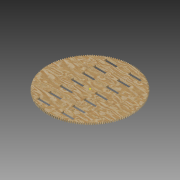
# Autodesk Inventor part: 1228_Major Gear_V1
Saved by Autodesk Inventor 2020 (Build 240168000, 168)
## iProperties
Created: 2019-09-12
Part Number: 1228_Major Gear_V1
Material: Generic
Document SubType Name: Modeling
Designer: MPI
Density: 1 g/cm^3
Appearance: Plywood - Weathered
Mass: 13454.9 g
Surface Area: 16406.6 cm^2
Volume: 13454.9 cm^3
Author: MPI
Autodesk Inventor part; units mm, degrees
sketch "Sketch1" plane through (0, 0, 0) normal (0, 0, 1) x (1, 0, 0)
  circle A0 centre (0, 0) radius 525
  line L0 (120, 632.0408) -> (120, -573) construction
  circle A1 centre (0, 0) radius 475 construction
  circle A2 centre (-120, 459.5922) radius 4
  circle A3 centre (120, 459.5922) radius 4
  circle A4 centre (120, -459.5922) radius 4
  circle A5 centre (-120, -459.5922) radius 4
  line L1 (-121, 95) -> (187, 95) construction
  line L2 (-126, -95) -> (139, -95) construction
  circle A6 centre (120, 95) radius 4
  circle A7 centre (120, -95) radius 4
  circle A8 centre (-120, -95) radius 4
  line L3 (-120, -459.5922) -> (-120, 595) construction
  circle A9 centre (0, 0) radius 13
  line L4 (-270.1078, 305) -> (246.6178, 305) construction
  line L5 (-227.3021, -305) -> (263.4344, -305) construction
  circle A10 centre (120, 305) radius 4
  circle A11 centre (-120, 305) radius 4
  circle A12 centre (-120, 95) radius 4
  circle A13 centre (-120, -305) radius 4
  circle A14 centre (120, -305) radius 4
  dimension "d0" = 1050
  dimension "d6" = 950
  dimension "d29" = 120
  dimension "d52" = 190
  dimension "d53" = 95
  dimension "d69" = 240
  dimension "d75" = 26
  dimension "d84" = 210
  dimension "d85" = 210
  dimension "d86" = 8
  dimension "d87" = 8
  dimension "d88" = 8
  dimension "d89" = 8
  dimension "d90" = 8
  dimension "d91" = 8
  constraints: 20 point on line, 15 centre point, 12 end point, 6 equal radius, 5 point on circle, 3 horizontal, 2 coincident, 1 parallel
  measures "d0" diameter of A0
  measures "d6" diameter of A1
  measures "d29" distance from line of point (0, 0) L3
  measures "d52" distance between parallel lines of L2 L1
  measures "d53" distance from line of point (0, 0) L1
  measures "d69" distance between parallel lines of L0 L3
  measures "d75" diameter of A9
  measures "d84" distance between parallel lines of L4 L1
  measures "d85" distance between parallel lines of L5 L2
  measures "d86" diameter of A2
  measures "d87" diameter of A10
  measures "d88" diameter of A11
  measures "d89" diameter of A12
  measures "d90" diameter of A13
  measures "d91" diameter of A14
extrude "Extrusion8" add sketch "Sketch1" along normal blind 19.05
sketch "Sketch4" plane through (0, 0, 19.05) normal (0, 0, 1) x (1, 0, 0)
  point P0 (0, 0)
spur gear teeth "Spur Gear2" teeth 168 pitch diameter 1008 tip diameter 1016 root diameter 989.0539 face width 20 trims to tip circle yes start plane through (0, 0, 19.05) normal (0, 0, 1) x (1, 0, 0)
sketch "Sketch5" plane through (0, 0, 19.05) normal (0, 0, 1) x (1, 0, 0)
  line L0 (74, 608.4937) -> (74, -743.4634) construction
  line L1 (214, 16) -> (74, 16)
  line L2 (74, 16) -> (74, -16)
  line L3 (74, -16) -> (214, -16)
  line L4 (214, -16) -> (214, 16)
  line L5 (263.9266, -151) -> (-273.4398, -151) construction
  line L6 (263.9266, -286) -> (-279.3841, -286) construction
  line L7 (263.9266, -421) -> (-273.4398, -421) construction
  line L8 (286.5207, 151) -> (-235.3905, 151) construction
  line L9 (278.1986, 286) -> (-235.3905, 286) construction
  line L10 (278.1986, 421) -> (-222.313, 421) construction
  line L11 (216, 20) -> (72, 20)
  line L12 (70, 18) -> (70, -18)
  line L13 (72, -20) -> (216, -20)
  line L14 (218, -18) -> (218, 18)
  arc A0 (218, 18) -> (216, 20) centre (216, 18) ccw
  arc A1 (216, -20) -> (218, -18) centre (216, -18) ccw
  arc A2 (72, 20) -> (70, 18) centre (72, 18) ccw
  arc A3 (70, -18) -> (72, -20) centre (72, -18) ccw
  line L15 (216, -115) -> (72, -115)
  line L16 (70, -117) -> (70, -153)
  line L17 (72, -155) -> (216, -155)
  line L18 (218, -153) -> (218, -117)
  arc A4 (218, -117) -> (216, -115) centre (216, -117) ccw
  arc A5 (216, -155) -> (218, -153) centre (216, -153) ccw
  arc A6 (72, -115) -> (70, -117) centre (72, -117) ccw
  arc A7 (70, -153) -> (72, -155) centre (72, -153) ccw
  line L19 (216, -250) -> (72, -250)
  line L20 (70, -252) -> (70, -288)
  line L21 (72, -290) -> (216, -290)
  line L22 (218, -288) -> (218, -252)
  arc A8 (218, -252) -> (216, -250) centre (216, -252) ccw
  arc A9 (216, -290) -> (218, -288) centre (216, -288) ccw
  arc A10 (72, -250) -> (70, -252) centre (72, -252) ccw
  arc A11 (70, -288) -> (72, -290) centre (72, -288) ccw
  line L23 (216, -385) -> (72, -385)
  line L24 (70, -387) -> (70, -423)
  line L25 (72, -425) -> (216, -425)
  line L26 (218, -423) -> (218, -387)
  arc A12 (218, -387) -> (216, -385) centre (216, -387) ccw
  arc A13 (216, -425) -> (218, -423) centre (216, -423) ccw
  arc A14 (72, -385) -> (70, -387) centre (72, -387) ccw
  arc A15 (70, -423) -> (72, -425) centre (72, -423) ccw
  line L27 (216, 155) -> (72, 155)
  line L28 (70, 153) -> (70, 117)
  line L29 (72, 115) -> (216, 115)
  line L30 (218, 117) -> (218, 153)
  arc A16 (218, 153) -> (216, 155) centre (216, 153) ccw
  arc A17 (216, 115) -> (218, 117) centre (216, 117) ccw
  arc A18 (72, 155) -> (70, 153) centre (72, 153) ccw
  arc A19 (70, 117) -> (72, 115) centre (72, 117) ccw
  line L31 (216, 290) -> (72, 290)
  line L32 (70, 288) -> (70, 252)
  line L33 (72, 250) -> (216, 250)
  line L34 (218, 252) -> (218, 288)
  arc A20 (218, 288) -> (216, 290) centre (216, 288) ccw
  arc A21 (216, 250) -> (218, 252) centre (216, 252) ccw
  arc A22 (72, 290) -> (70, 288) centre (72, 288) ccw
  arc A23 (70, 252) -> (72, 250) centre (72, 252) ccw
  line L35 (216, 425) -> (72, 425)
  line L36 (70, 423) -> (70, 387)
  line L37 (72, 385) -> (216, 385)
  line L38 (218, 387) -> (218, 423)
  arc A24 (218, 423) -> (216, 425) centre (216, 423) ccw
  arc A25 (216, 385) -> (218, 387) centre (216, 387) ccw
  arc A26 (72, 425) -> (70, 423) centre (72, 423) ccw
  arc A27 (70, 387) -> (72, 385) centre (72, 387) ccw
  circle A28 centre (0, 0) radius 13 projected
  line L39 (0, 0) -> (0, -697.8979)
  line L40 (-216, 20) -> (-72, 20)
  line L41 (-70, 18) -> (-70, -18)
  line L42 (-72, -20) -> (-216, -20)
  line L43 (-218, -18) -> (-218, 18)
  arc A29 (-216, 20) -> (-218, 18) centre (-216, 18) ccw
  arc A30 (-218, -18) -> (-216, -20) centre (-216, -18) ccw
  arc A31 (-70, 18) -> (-72, 20) centre (-72, 18) ccw
  arc A32 (-72, -20) -> (-70, -18) centre (-72, -18) ccw
  line L44 (-218, -153) -> (-218, -117)
  line L45 (-72, -155) -> (-216, -155)
  line L46 (-216, -115) -> (-72, -115)
  arc A33 (-72, -155) -> (-70, -153) centre (-72, -153) ccw
  arc A34 (-70, -117) -> (-72, -115) centre (-72, -117) ccw
  arc A35 (-218, -153) -> (-216, -155) centre (-216, -153) ccw
  arc A36 (-216, -115) -> (-218, -117) centre (-216, -117) ccw
  line L47 (-70, -117) -> (-70, -153)
  line L48 (-218, -288) -> (-218, -252)
  line L49 (-72, -290) -> (-216, -290)
  line L50 (-216, -250) -> (-72, -250)
  arc A37 (-72, -290) -> (-70, -288) centre (-72, -288) ccw
  arc A38 (-70, -252) -> (-72, -250) centre (-72, -252) ccw
  arc A39 (-218, -288) -> (-216, -290) centre (-216, -288) ccw
  arc A40 (-216, -250) -> (-218, -252) centre (-216, -252) ccw
  line L51 (-70, -252) -> (-70, -288)
  line L52 (-218, -423) -> (-218, -387)
  line L53 (-72, -425) -> (-216, -425)
  line L54 (-216, -385) -> (-72, -385)
  arc A41 (-72, -425) -> (-70, -423) centre (-72, -423) ccw
  arc A42 (-70, -387) -> (-72, -385) centre (-72, -387) ccw
  arc A43 (-218, -423) -> (-216, -425) centre (-216, -423) ccw
  arc A44 (-216, -385) -> (-218, -387) centre (-216, -387) ccw
  line L55 (-70, -387) -> (-70, -423)
  line L56 (-218, 117) -> (-218, 153)
  line L57 (-216, 155) -> (-72, 155)
  arc A45 (-218, 117) -> (-216, 115) centre (-216, 117) ccw
  line L58 (-72, 115) -> (-216, 115)
  arc A46 (-216, 155) -> (-218, 153) centre (-216, 153) ccw
  arc A47 (-70, 153) -> (-72, 155) centre (-72, 153) ccw
  line L59 (-70, 153) -> (-70, 117)
  arc A48 (-72, 115) -> (-70, 117) centre (-72, 117) ccw
  line L60 (-218, 252) -> (-218, 288)
  line L61 (-216, 290) -> (-72, 290)
  arc A49 (-218, 252) -> (-216, 250) centre (-216, 252) ccw
  line L62 (-72, 250) -> (-216, 250)
  arc A50 (-216, 290) -> (-218, 288) centre (-216, 288) ccw
  arc A51 (-70, 288) -> (-72, 290) centre (-72, 288) ccw
  line L63 (-70, 288) -> (-70, 252)
  arc A52 (-72, 250) -> (-70, 252) centre (-72, 252) ccw
  line L64 (-218, 387) -> (-218, 423)
  line L65 (-216, 425) -> (-72, 425)
  arc A53 (-218, 387) -> (-216, 385) centre (-216, 387) ccw
  line L66 (-72, 385) -> (-216, 385)
  arc A54 (-216, 425) -> (-218, 423) centre (-216, 423) ccw
  arc A55 (-70, 423) -> (-72, 425) centre (-72, 423) ccw
  line L67 (-70, 423) -> (-70, 387)
  arc A56 (-72, 385) -> (-70, 387) centre (-72, 387) ccw
  point P0 (-214, 16)
  point P1 (-74, -16)
  point P2 (-74, 16)
  point P3 (-214, -16)
  dimension "d92" = 74
  dimension "d94" = 32
  dimension "d95" = 16
  dimension "d96" = 135
  dimension "d97" = 135
  dimension "d98" = 135
  dimension "d99" = 135
  dimension "d100" = 135
  dimension "d101" = 135
  dimension "d102" = 140
  dimension "d103" = 0
  dimension "d104" = 4
  dimension "d105" = 2
  dimension "d106" = 2
  dimension "d107" = 2
  dimension "d108" = 2
  dimension "d109" = 2
  dimension "d110" = 2
  dimension "d111" = 2
  dimension "d112" = 2
  dimension "d113" = 2
  dimension "d114" = 2
  dimension "d115" = 2
  dimension "d116" = 2
  dimension "d117" = 2
  dimension "d118" = 2
  dimension "d119" = 2
  dimension "d120" = 2
  dimension "d121" = 2
  dimension "d122" = 2
  dimension "d123" = 2
  dimension "d124" = 2
  dimension "d125" = 2
  constraints: 136 end point, 112 point on circle, 88 symmetric about line, 56 centre point, 56 tangent, 16 parallel, 11 collinear, 8 perpendicular, 7 equal radius, 7 horizontal, 4 vertical, 31 other
  measures "d92" distance from line of point (0, 0) L0
  measures "d94" distance of L3.end L1.start
  measures "d95" distance from line of point (0, 0) L3
  measures "d96" distance between parallel lines of L5 L3
  measures "d97" distance between parallel lines of L6 L5
  measures "d98" distance between parallel lines of L7 L6
  measures "d99" distance between parallel lines of L8 L1
  measures "d100" distance between parallel lines of L9 L8
  measures "d101" distance between parallel lines of L10 L9
  measures "d102" distance of L2.end L3.end
  measures "d103" distance between parallel lines of L0 L2
  measures "d104" distance between parallel lines of L4 L14
  measures "d105" radius of A0
  measures "d106" radius of A2
  measures "d107" radius of A3
  measures "d108" radius of A4
  measures "d109" radius of A6
  measures "d110" radius of A7
  measures "d111" radius of A8
  measures "d112" radius of A10
  measures "d113" radius of A11
  measures "d114" radius of A12
  measures "d115" radius of A14
  measures "d116" radius of A15
  measures "d117" radius of A16
  measures "d118" radius of A18
  measures "d119" radius of A19
  measures "d120" radius of A20
  measures "d121" radius of A22
  measures "d122" radius of A23
  measures "d123" radius of A24
  measures "d124" radius of A26
  measures "d125" radius of A27
extrude "Extrusion9" cut sketch "Sketch5" against normal through all contours L4 L3 L2 L1 | A0 L14 A1 L13 A3 L12 A2 L11 | A4 L18 A5 L17 A7 L16 A6 L15 | A8 L22 A9 L21 A11 L20 A10 L19 | A12 L26 A13 L25 A15 L24 A14 L23 | A16 L30 A17 L29 A19 L28 A18 L27 | A20 L34 A21 L33 A23 L32 A22 L31 | A24 L38 A25 L37 A27 L36 A26 L35 | L40 A31 L41 A32 L42 A30 L43 A29 | L44 A36 L46 A34 L47 A33 L45 A35 | L48 A40 L50 A38 L51 A37 L49 A39 | L52 A44 L54 A42 L55 A41 L53 A43 | L56 A46 L57 A47 L59 A48 L58 A45 | L60 A50 L61 A51 L63 A52 L62 A49 | L64 A54 L65 A55 L67 A56 L66 A53
ref_plane "Work Plane1" through (0, 0, 12.85) normal (0, 0, 1) x (1, 0, 0)
sketch "Sketch7" plane through (0, 0, 12.85) normal (0, 0, 1) x (1, 0, 0)
  circle A0 centre (-120, -459.5922) radius 4 projected
  circle A1 centre (-120, -459.5922) radius 4
  point P0 (0, 0)
  point P1 (-120, -305)
  point P2 (-120, -95)
  point P3 (-120, 95)
  constraints: 1 centre point, 1 coincident
sketch "Sketch8" plane through (0, 0, 19.05) normal (0, 0, 1) x (1, 0, 0)
  circle A0 centre (-120, -459.5922) radius 4 projected
  circle A1 centre (-120, -459.5922) radius 8.5
  point P0 (0, 0)
  dimension "d131" = 17
  constraints: 1 centre point, 1 coincident
  measures "d131" diameter of A1
loft "Loft1" cut profiles "Sketch7", "Sketch8" contours all / A0 | A1
pattern_linear "Rectangular Pattern1" count 2 spacing 154.58 along (0, 1, 0) of "Loft1"
pattern_linear "Rectangular Pattern2" count 2 spacing 364.585 along (0, 1, 0) of "Loft1"
ref_plane "Work Plane2" through (-216, 0, 19.05) normal (0, 1, 0) x (1, 0, 0)
mirror "Mirror1" about plane through (-216, 0, 19.05) normal (0, 1, 0) of "Loft1", "Rectangular Pattern1", "Rectangular Pattern2"
ref_plane "Work Plane3" through (0, 387, 19.05) normal (-1, 0, 0) x (0, 0, 1)
mirror "Mirror2" about plane through (0, 387, 19.05) normal (-1, 0, 0) of "Loft1", "Rectangular Pattern1", "Rectangular Pattern2", "Mirror1"
sketch "Sketch9" plane through (0, 0, 0) normal (0, 0, -1) x (-1, 0, 0)
  circle A0 centre (0, 0) radius 13 projected
  circle A1 centre (0, 0) radius 25.4
  dimension "d142" = 50.8
  constraints: 1 centre point, 1 coincident
  measures "d142" diameter of A1
extrude "Extrusion11" cut sketch "Sketch9" against normal blind 13 contours A0 | A1
body "Solid8"
